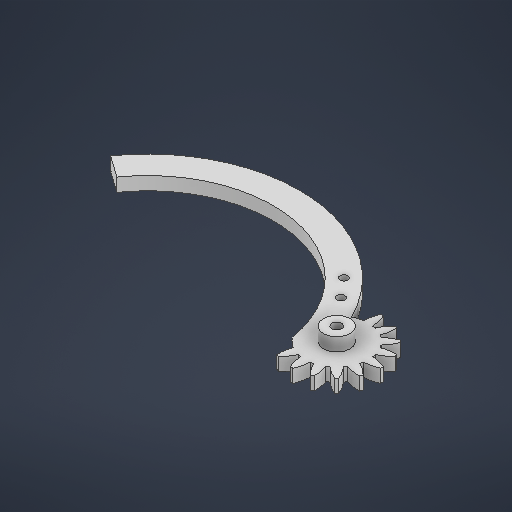
# Autodesk Inventor part: Left_Top_Gripper
Saved by Autodesk Inventor 2026.1 (Build 301233020, 233B)
## iProperties
Created: 2025-10-15
Part Number: Left_Top_Gripper
Material: Generic
Document SubType Name: Modeling
Designer: Garfieldcmix
Density: 1 g/cm^3
Appearance: Default
Author: Garfieldcmix
Autodesk Inventor part; units mm, degrees
ref_plane "YZ Plane" through (0, 0, 0) normal (1, 0, 0) x (0, 1, 0)
ref_plane "XZ Plane" through (0, 0, 0) normal (0, 1, 0) x (-1, 0, 0)
ref_plane "XY Plane" through (0, 0, 0) normal (0, 0, 1) x (1, 0, 0)
derived "Left_Bottom_Gripper.ipt"
sketch "Sketch1" plane through (0, 0, 0) normal (0, 1, 0) x (-1, 0, 0)
  arc A0 (-44.6354, -16.246) -> (38.9097, -27.2449) centre (0, 0) ccw
  line L0 (-44.6354, -16.246) -> (-54.0323, -19.6662)
  line L1 (38.9097, -27.2449) -> (47.1012, -32.9806)
  arc A1 (-54.0323, -19.6662) -> (47.1012, -32.9806) centre (0, 0) ccw
  line L2 (0, -76.3984) -> (0, 12.7331) construction
extrude "Extrusion1" add sketch "Sketch1" along normal blind 5
sketch "Sketch5" plane through (0, 0, 0) normal (0, 1, 0) x (-1, 0, 0)
  arc A0 (-46.8208, -8.0042) -> (-44.6354, -16.246) centre (-56.5705, -15) ccw
  line L0 (60.9407, 0) -> (-93.2763, 0) construction
  line L1 (-44.6354, -16.246) -> (-54.0323, -19.6662) construction
  arc A1 (-44.6354, -16.246) -> (38.9097, -27.2449) centre (0, 0) ccw construction
  arc A2 (-46.8208, -8.0042) -> (-44.6354, -16.246) centre (0, 0) ccw
  circle A3 centre (-56.5705, -15) radius 3
  dimension "d3" = 24
  dimension "d4" = 15
  dimension "d25" = 6
  constraints: 5 point on circle, 3 centre point, 1 coincident, 1 concentric, 1 end point
  measures "d3" diameter of A0
  measures "d4" distance from line of A0.centre L0
  measures "d25" diameter of A3
extrude "Extrusion2" add sketch "Sketch5" along normal up to surface (5 mm away)
sketch "Sketch6" plane through (0, 0, 0) normal (0, 1, 0) x (-1, 0, 0)
  arc A0 (-46.8208, -8.0042) -> (-51.3777, -25.8182) centre (-56.5705, -15) ccw construction
  line L0 (-56.5705, -15) -> (-56.5705, -3) construction
  line L1 (-54.8205, -3.1283) -> (-58.3205, -3.1283)
  line L2 (-58.3205, -3.1283) -> (-57.0955, 2.1217) construction
  line L3 (-54.8205, -3.1283) -> (-56.0455, 2.1217) construction
  line L4 (-56.0455, 2.1217) -> (-57.0955, 2.1217)
  arc A1 (-54.8205, -3.1283) -> (-56.0455, 2.1217) centre (-68.8117, -3.625) ccw
  arc A2 (-57.0955, 2.1217) -> (-58.3205, -3.1283) centre (-44.3294, -3.625) ccw
  point P0 (0, 0)
  dimension "d13" = 3.5
  dimension "d14" = 1.05
  dimension "d15" = 5.25
  dimension "d16" = 14
  constraints: 10 end point, 7 point on circle, 2 centre point, 1 equal radius, 1 horizontal, 1 symmetric about line, 1 vertical
  measures "d13" distance of L1.start L1.end
  measures "d14" distance of L3.end L2.end
  measures "d15" vertical distance of L3.end L1.start
  measures "d16" radius of A1
extrude "Extrusion3" add sketch "Sketch6" along normal up to surface (5 mm away)
pattern_circular "Circular Pattern1" count 2 over 22.5 about axis through (56.5705, 0, -15) along (0, -1, 0) of "Extrusion3"
pattern_circular "Circular Pattern3" count 9 over 180 about axis through (56.5705, 0, -15) along (0, 1, 0) of "Extrusion3"
sketch "Sketch7" plane through (-47.1012, 5, -32.9806) normal (0, 1, 0) x (0.819152, 0, 0.5735764)
  circle A0 centre (75.4561, 49.3339) radius 1.5 projected
  circle A1 centre (66.6165, 51.7024) radius 1.5 projected
  point P0 (57.5, 0)
extrude "Extrusion4" cut sketch "Sketch7" against normal up to surface (5 mm away)
sketch "Sketch8" plane through (-47.1012, 5, -32.9806) normal (0, 1, 0) x (0.819152, 0, 0.5735764)
  circle A0 centre (95.2362, 44.7348) radius 3 construction
  circle A1 centre (95.2362, 44.7348) radius 5
  circle A2 centre (95.2362, 44.7348) radius 1.85
  point P0 (57.5, 0)
  dimension "d31" = 10
  dimension "d34" = 3.7
  constraints: 2 centre point, 2 coincident
  measures "d31" diameter of A1
  measures "d34" diameter of A2
extrude "Extrusion5" add sketch "Sketch8" along normal blind 5
sketch "Sketch3" plane through (0, 17, 0) normal (0, 1, 0) x (1, 0, 0)
  circle A0 centre (43.0055, 30.1128) radius 1.5 projected
  arc A1 (44.6354, 16.246) -> (30.5324, 36.3871) centre (0, 0) ccw construction
  arc A2 (54.0323, 19.6662) -> (36.9603, 44.0476) centre (0, 0) ccw construction
  line L0 (44.6354, 16.246) -> (54.0323, 19.6662) construction
  line L1 (36.9603, 44.0476) -> (30.5324, 36.3871) construction
  line L2 (38.9097, 27.2449) -> (47.1012, 32.9806) construction
  line L3 (33.5876, 33.5876) -> (40.6586, 40.6586) construction
  circle A3 centre (37.1231, 37.1231) radius 1.5 projected
body "Solid1"
